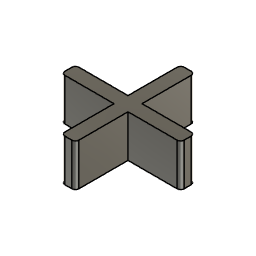
Plus (Autodesk Fusion 360 design; units mm, degrees)
Autodesk Fusion 360 part; units mm, degrees
sketch "スケッチ1" plane through (0, 0, 0) normal (0, 0, 1) x (1, 0, 0)
  line L0 (-200, 200) -> (200, 200) construction
  line L1 (200, 200) -> (200, -200) construction
  line L2 (200, -200) -> (-200, -200) construction
  line L3 (-200, -200) -> (-200, 200) construction
  line L4 (-200, 200) -> (200, -200) construction
  line L5 (200, 200) -> (-200, -200) construction
  line L6 (-200, 200) -> (-1600, 200)
  line L7 (-1700, 100) -> (-1700, -100)
  line L8 (-1600, -200) -> (-200, -200)
  arc A0 (-1600, 200) -> (-1700, 100) centre (-1600, 100) ccw
  arc A1 (-1700, -100) -> (-1600, -200) centre (-1600, -100) ccw
  line L9 (-100, -1700) -> (100, -1700)
  arc A2 (-200, -1600) -> (-100, -1700) centre (-100, -1600) ccw
  arc A3 (100, -1700) -> (200, -1600) centre (100, -1600) ccw
  line L10 (200, -1600) -> (200, -200)
  line L11 (-200, -200) -> (-200, -1600)
  line L12 (1700, -100) -> (1700, 100)
  arc A4 (1600, -200) -> (1700, -100) centre (1600, -100) ccw
  arc A5 (1700, 100) -> (1600, 200) centre (1600, 100) ccw
  line L13 (1600, 200) -> (200, 200)
  line L14 (200, -200) -> (1600, -200)
  line L15 (100, 1700) -> (-100, 1700)
  arc A6 (200, 1600) -> (100, 1700) centre (100, 1600) ccw
  arc A7 (-100, 1700) -> (-200, 1600) centre (-100, 1600) ccw
  line L16 (-200, 1600) -> (-200, 200)
  line L17 (200, 200) -> (200, 1600)
  dimension "d1" = 100
  dimension "d2" = 400
  dimension "d3" = 1500
  dimension "d5" = 360
  constraint horizontal L0
  constraint perpendicular L0 L1
  constraint parallel L0 L2
  constraint parallel L1 L3
  constraint coincident L4 origin
  constraint coincident L5 origin
  constraint perpendicular L3 L6
  constraint perpendicular L6 L7
  constraint perpendicular L3 L8
  constraint tangent L6 A0
  constraint tangent L7 A0
  constraint tangent L7 A1
  constraint tangent L8 A1
  constraint equal A0 A1
  constraint equal L0 L3
  measures "d1" radius of A0
  measures "d2" distance of L6.end L8.start
  measures "d3" distance of L3 L7.start
extrude "押し出し1" add sketch "スケッチ1" along normal blind 1200
